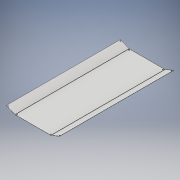
# Autodesk Inventor part: sideplate part 4
Saved by Autodesk Inventor 2018 (Build 220112000, 112)
## iProperties
Created: 2018-06-15
Part Number: sideplate part 4
Material: Generic
Document SubType Name: Sheet Metal
Designer: John Viljoen
Density: 1 g/cm^3
Sheet Metal Rule: Default_mm
Appearance: Default
Flat Pattern Width: 17.41 cm
Flat Pattern Length: 36.287 cm
Flat Pattern Area: 631.755 cm^2
Sheet Metal Width: 174.100 mm
Sheet Metal Length: 362.870 mm
Sheet Metal Area: 63175.525 mm^2
Author: John Viljoen
Autodesk Inventor part; units mm, degrees
ref_plane "YZ Plane" through (0, 0, 0) normal (1, 0, 0) x (0, 1, 0)
ref_plane "XZ Plane" through (0, 0, 0) normal (0, 1, 0) x (-1, 0, 0)
ref_plane "XY Plane" through (0, 0, 0) normal (0, 0, 1) x (1, 0, 0)
sketch "Sketch1" plane through (0, 0, 0) normal (0, 0, 1) x (1, 0, 0)
  line L0 (0, 0) -> (113.5, 0)
  line L1 (113.5, 0) -> (113.5, 338.525)
  line L2 (113.5, 338.525) -> (0, 338.525)
  line L3 (0, 338.525) -> (0, 0)
  dimension "d0" = 113.5
  dimension "d1" = 338.525
  measures "d0" distance of L2.end L1.end
  measures "d1" distance of L1.end L0.end
extrude "Plate1" add sketch "Sketch1" along normal blind 0.5
sketch "Sketch2" plane through (114.0764, 338.525, 0.6152) normal (0.3842953, 0, -0.9232102) x (0, 1, 0)
  line L0 (-338.525, 0) -> (0, 0)
  line L1 (0, 0) -> (0, 29.6214)
  line L2 (0, 29.6214) -> (-338.525, 29.6214)
  line L3 (-338.525, 29.6214) -> (-338.525, 0)
  constraints: 6 end point, 1 horizontal, 1 perpendicular, 1 vertical
edge flange "Flange1" height 30.021 angle 22.6 thickness 0.5 bend radius 1.5 thickness toward (0.3842953, 0, -0.9232102) relief straight relief width 0.5 relief depth 0.25 edges at (113.5, 169.2625, 0.5) wall of the first edge with corners at (114.0764, 0, 0.6152) (114.0764, 338.525, 0.6152) (141.4232, 338.525, 11.9985) (141.4232, 0, 11.9985)
bend "Bend1"
corner "Corner1"
sketch "Sketch3" plane through (-0.5764, 0, 0.6152) normal (-0.3842953, 0, -0.9232102) x (0, -1, 0)
  line L0 (-338.525, 0) -> (0, 0)
  line L1 (0, 0) -> (0, 29.6214)
  line L2 (0, 29.6214) -> (-338.525, 29.6214)
  line L3 (-338.525, 29.6214) -> (-338.525, 0)
  constraints: 6 end point, 1 horizontal, 1 perpendicular, 1 vertical
edge flange "Flange2" height 30.021 angle 22.6 thickness 0.5 bend radius 1.5 thickness toward (-0.3842953, 0, -0.9232102) relief straight relief width 0.5 relief depth 0.25 edges at (0, 169.2625, 0.5) wall of the first edge with corners at (-0.5764, 338.525, 0.6152) (-0.5764, 0, 0.6152) (-27.9232, 0, 11.9985) (-27.9232, 338.525, 11.9985)
bend "Bend2"
corner "Corner2"
sketch "Sketch4" plane through (-27.9232, 0, 11.9985) normal (0.3842953, 0, 0.9232102) x (0.9232102, 0, -0.3842953)
  line L0 (0, 338.525) -> (0, 0) projected
  line L1 (0, 338.525) -> (0, 335.35) construction
  line L2 (0, 335.35) -> (3.175, 335.35) construction
  circle A0 centre (3.175, 335.35) radius 1.25
  line L3 (0, 0) -> (0, 3.175) construction
  line L4 (0, 3.175) -> (3.175, 3.175) construction
  line L5 (3.175, 3.175) -> (3.175, 3.35) construction
  circle A1 centre (3.175, 3.35) radius 1.25
  point P0 (30.39, 0)
  dimension "d23" = 3.175
  dimension "d24" = 3.175
  dimension "d25" = 2.5
  dimension "d26" = 3.175
  dimension "d27" = 3.175
  dimension "d62" = 0.175
  dimension "d63" = 2.5
  constraints: 10 end point, 3 coincident, 2 centre point, 2 perpendicular, 2 point on line, 1 vertical
  measures "d23" distance of L0.start L1.end
  measures "d24" distance of L1.end L2.end
  measures "d25" diameter of A0
  measures "d26" distance of L0.end L3.end
  measures "d27" distance of L3.end L4.end
  measures "d62" distance of L5.start L5.end
  measures "d63" diameter of A1
extrude "Extrusion1" cut sketch "Sketch4" against normal blind 10
sketch "Sketch5" plane through (0, 0, 0.5) normal (0, 0, 1) x (1, 0, 0)
  line L0 (0, 0) -> (0, 338.525) projected
  line L1 (113.5, 0) -> (0, 0) projected
  line L2 (113.5, 338.525) -> (113.5, 0) projected
  line L3 (0, 338.525) -> (0, 335.35) construction
  line L4 (0, 335.35) -> (3.175, 335.35) construction
  line L5 (113.5, 338.525) -> (113.5, 335.35) construction
  line L6 (113.5, 335.35) -> (110.325, 335.35) construction
  line L7 (0, 0) -> (3.175, 0) construction
  line L8 (0, 0) -> (113.5, 0) construction
  line L9 (3.175, 0) -> (3.175, 3.175) construction
  line L10 (113.5, 0) -> (113.5, 3.175) construction
  line L11 (113.5, 3.175) -> (110.325, 3.175) construction
  circle A0 centre (3.175, 335.35) radius 1.25
  circle A1 centre (110.325, 335.35) radius 1.25
  line L12 (3.175, 3.175) -> (3.175, 3.35) construction
  line L13 (110.325, 3.175) -> (110.325, 3.35) construction
  circle A2 centre (110.325, 3.35) radius 1.25
  circle A3 centre (3.175, 3.35) radius 1.25
  dimension "d31" = 3.175
  dimension "d32" = 3.175
  dimension "d33" = 3.175
  dimension "d34" = 3.175
  dimension "d35" = 3.175
  dimension "d36" = 3.175
  dimension "d37" = 3.175
  dimension "d38" = 3.175
  dimension "d41" = 2.5
  dimension "d42" = 2.5
  dimension "d58" = 0.175
  dimension "d59" = 0.175
  dimension "d60" = 2.5
  dimension "d61" = 2.5
  constraints: 20 end point, 6 coincident, 4 centre point, 4 perpendicular, 4 point on line, 2 vertical
  measures "d31" distance of L0.end L3.end
  measures "d32" distance of L3.end L4.end
  measures "d33" distance of L2.start L5.end
  measures "d34" distance of L5.end L6.end
  measures "d35" distance of L0.start L7.end
  measures "d36" distance of L7.end L9.end
  measures "d37" distance of L1.start L10.end
  measures "d38" distance of L10.end L11.end
  measures "d41" diameter of A0
  measures "d42" diameter of A1
  measures "d58" distance of L12.start L12.end
  measures "d59" distance of L13.start L13.end
  measures "d60" diameter of A2
  measures "d61" diameter of A3
extrude "Extrusion2" cut sketch "Sketch5" against normal blind 10
sketch "Sketch6" plane through (141.4232, 0, 11.9985) normal (-0.3842953, 0, 0.9232102) x (0.9232102, 0, 0.3842953)
  line L0 (0, 338.525) -> (0, 335.35) construction
  line L1 (0, 0) -> (0, 338.525) construction
  line L2 (0, 335.35) -> (-3.175, 335.35) construction
  line L3 (0, 0) -> (0, 3.175) construction
  line L4 (0, 3.175) -> (-3.175, 3.175) construction
  circle A0 centre (-3.175, 335.35) radius 1.25
  line L5 (-3.175, 3.175) -> (-3.175, 3.35) construction
  circle A1 centre (-3.175, 3.35) radius 1.25
  point P0 (-135.1743, 0)
  dimension "d45" = 3.175
  dimension "d46" = 3.175
  dimension "d47" = 3.175
  dimension "d48" = 3.175
  dimension "d50" = 2.5
  dimension "d64" = 0.175
  dimension "d65" = 2.5
  constraints: 10 end point, 3 coincident, 2 centre point, 2 perpendicular, 2 point on line, 1 vertical
  measures "d45" distance of L0.start L0.end
  measures "d46" distance of L0.end L2.end
  measures "d47" distance of L1.start L3.end
  measures "d48" distance of L3.end L4.end
  measures "d50" diameter of A0
  measures "d64" distance of L5.start L5.end
  measures "d65" diameter of A1
extrude "Extrusion3" cut sketch "Sketch6" against normal blind 10
sketch "Sketch7" plane through (0, 0, 0.5) normal (0, 0, 1) x (1, 0, 0)
  line L0 (-71.3896, 0) -> (266.456, 0)
  line L1 (266.456, 0) -> (266.456, 0.175)
  line L2 (266.456, 0.175) -> (-71.3896, 0.175)
  line L3 (-71.3896, 0.175) -> (-71.3896, 0)
  dimension "d53" = 0.175
  constraints: 8 end point, 2 parallel, 1 horizontal, 1 perpendicular
  measures "d53" distance of L1.end L0.end
extrude "Extrusion4" cut sketch "Sketch7" against normal blind 100 and the other way blind 100
sketch "Sketch9" plane through (-28.1153, 338.525, 11.5369) normal (0, 1, 0) x (0.9232102, 0, -0.3842953)
  line L0 (29.6214, -0.5) -> (29.6214, 0) projected
  line L1 (29.6214, 0) -> (0, 0) projected
  line L2 (0, -0.5) -> (0, 0) projected
  line L3 (0, -0.5) -> (29.6214, -0.5) projected
  point P0 (30.39, -0.1536)
extrude "Extrusion5" add sketch "Sketch9" along normal blind 30.87
sketch "Sketch10" plane through (0, 338.525, 0.5) normal (0, 1, 0) x (1, 0, 0)
  line L0 (-0.5764, -0.1152) -> (-0.7686, 0.3464) projected
  arc A0 (0, 0) -> (-0.5764, -0.1152) centre (0, -1.5) ccw projected
  line L1 (0, 0.5) -> (0, 0) projected
  arc A1 (0, 0.5) -> (-0.7686, 0.3464) centre (0, -1.5) ccw projected
extrude "Extrusion6" add sketch "Sketch10" along normal blind 30.87
sketch "Sketch11" plane through (0, 338.525, 0) normal (0, 1, 0) x (1, 0, 0)
  line L0 (0, -0.5) -> (113.5, -0.5) projected
  line L1 (113.5, 0) -> (113.5, -0.5) projected
  line L2 (113.5, 0) -> (0, 0) projected
  line L3 (0, 0) -> (0, -0.5) projected
extrude "Extrusion7" add sketch "Sketch11" along normal blind 30.87
sketch "Sketch12" plane through (113.5, 338.525, 0.5) normal (0, 1, 0) x (1, 0, 0)
  line L0 (0.7686, 0.3464) -> (0.5764, -0.1152) projected
  arc A0 (0.7686, 0.3464) -> (0, 0.5) centre (0, -1.5) ccw projected
  line L1 (0, 0.5) -> (0, 0) projected
  arc A1 (0.5764, -0.1152) -> (0, 0) centre (0, -1.5) ccw projected
  point P0 (-113.5, 0.5)
extrude "Extrusion8" add sketch "Sketch12" along normal blind 30.87
sketch "Sketch13" plane through (114.0764, 338.525, 0.6152) normal (0, 1, 0) x (0.9232102, 0, 0.3842953)
  line L0 (0, 0.5) -> (0, 0) projected
  line L1 (29.6214, 0) -> (0, 0) projected
  line L2 (29.6214, 0) -> (29.6214, 0.5) projected
  line L3 (29.6214, 0.5) -> (0, 0.5) projected
  point P0 (-105.553, -43.2711)
extrude "Extrusion9" add sketch "Sketch13" along normal blind 30.87
sketch "Sketch14" plane through (0, 0, 0.5) normal (0, 0, 1) x (1, 0, 0)
  circle A0 centre (3.175, 335.35) radius 1.25 projected
  point P0 (0, 0)
extrude "Extrusion10" add sketch "Sketch14" against normal up to surface (0.5 mm away)
sketch "Sketch15" plane through (0, 0, 0.5) normal (0, 0, 1) x (1, 0, 0)
  circle A0 centre (110.325, 335.35) radius 1.25 projected
  point P0 (0, 0)
extrude "Extrusion11" add sketch "Sketch15" against normal up to surface (0.5 mm away)
sketch "Sketch16" plane through (141.4232, 0.175, 11.9985) normal (-0.3842953, 0, 0.9232102) x (0.9232102, 0, 0.3842953)
  circle A0 centre (-3.175, 335.175) radius 1.25 projected
  point P0 (-135.1743, -0.175)
extrude "Extrusion12" add sketch "Sketch16" against normal up to surface (0.5 mm away)
sketch "Sketch17" plane through (-0.5764, 0.175, 0.6152) normal (0.3842953, 0, 0.9232102) x (0.9232102, 0, -0.3842953)
  circle A0 centre (-26.4464, 335.175) radius 1.25 projected
  point P0 (0.7686, -0.175)
extrude "Extrusion13" add sketch "Sketch17" against normal up to surface (0.5 mm away)
sketch "Sketch18" plane through (0, 0, 0.5) normal (0, 0, 1) x (1, 0, 0)
  line L0 (113.5, 0.175) -> (113.5, 369.395) projected
  line L1 (0, 0.175) -> (0, 369.395) projected
  line L2 (0, 369.395) -> (0, 359.87) construction
  line L3 (0, 359.87) -> (3.175, 359.87) construction
  circle A0 centre (3.175, 359.87) radius 1.5
  line L4 (113.5, 369.395) -> (113.5, 359.87) construction
  line L5 (113.5, 359.87) -> (110.325, 359.87) construction
  circle A1 centre (110.325, 359.87) radius 1.5
  point P0 (0, 0)
  dimension "d84" = 9.525
  dimension "d85" = 3.175
  dimension "d86" = 3
  dimension "d87" = 9.525
  dimension "d88" = 3.175
  dimension "d89" = 3
  constraints: 8 end point, 2 centre point, 2 coincident, 2 perpendicular, 2 point on line
  measures "d84" distance of L1.end L2.end
  measures "d85" distance of L2.end L3.end
  measures "d86" diameter of A0
  measures "d87" distance of L0.end L4.end
  measures "d88" distance of L4.end L5.end
  measures "d89" diameter of A1
extrude "Extrusion14" cut sketch "Sketch18" against normal blind 30.87
sketch "Sketch19" plane through (-0.5764, 0.175, 0.6152) normal (0.3842953, 0, 0.9232102) x (0.9232102, 0, -0.3842953)
  line L0 (-29.6214, 369.22) -> (-29.6214, 0) projected
  line L1 (-29.6214, 369.22) -> (-29.6214, 359.695) construction
  line L2 (-29.6214, 359.695) -> (-26.4464, 359.695) construction
  circle A0 centre (-26.4464, 359.695) radius 1.5
  point P0 (0.7686, -0.175)
  dimension "d92" = 9.525
  dimension "d93" = 3.175
  dimension "d94" = 3
  constraints: 4 end point, 1 centre point, 1 coincident, 1 perpendicular, 1 point on line
  measures "d92" distance of L0.start L1.end
  measures "d93" distance of L1.end L2.end
  measures "d94" diameter of A0
extrude "Extrusion15" cut sketch "Sketch19" against normal blind 30.87
sketch "Sketch20" plane through (141.4232, 0.175, 11.9985) normal (-0.3842953, 0, 0.9232102) x (0.9232102, 0, 0.3842953)
  line L0 (0, 0) -> (0, 369.22) projected
  line L1 (0, 369.22) -> (0, 359.695)
  line L2 (0, 359.695) -> (-3.175, 359.695)
  circle A0 centre (-3.175, 359.695) radius 1.5
  point P0 (-135.1743, -0.175)
  dimension "d97" = 9.525
  dimension "d98" = 3.175
  dimension "d99" = 3
  constraints: 4 end point, 1 centre point, 1 coincident, 1 perpendicular, 1 point on line
  measures "d97" distance of L0.end L1.end
  measures "d98" distance of L1.end L2.end
  measures "d99" diameter of A0
extrude "Extrusion16" cut sketch "Sketch20" against normal blind 30.87
sketch "Sketch21" plane through (0, 0, 0.5) normal (0, 0, 1) x (1, 0, 0)
  line L0 (-35.0424, 369.395) -> (185.2939, 369.395)
  line L1 (185.2939, 369.395) -> (185.2939, 363.045)
  line L2 (185.2939, 363.045) -> (-35.0424, 363.045)
  line L3 (-35.0424, 363.045) -> (-35.0424, 369.395)
  point P0 (0, 0)
  dimension "d102" = 6.35
  constraints: 8 end point, 2 parallel, 1 horizontal, 1 perpendicular
  measures "d102" distance of L0.end L1.end
extrude "Extrusion17" cut sketch "Sketch21" against normal blind 30.87 and the other way blind 15.435
equation "\"d2\" = Thickness"
equation "\"d3\" = BendReliefWidth"
equation "\"d4\" = BendReliefDepth"
equation "\"d5\" = MinimumRemnant"
equation "\"d6\" = TransitionRadius"
equation "\"d10\" = CornerReliefSize"
equation "\"d11\" = GapSize"
equation "\"d12\" = JacobiRadiusSize"
equation "\"d13\" = BendReliefWidth"
equation "\"d14\" = BendReliefDepth"
equation "\"d15\" = MinimumRemnant"
equation "\"d16\" = TransitionRadius"
equation "\"d20\" = CornerReliefSize"
equation "\"d21\" = GapSize"
equation "\"d22\" = JacobiRadiusSize"
equation "\"BendRadius\" = Thickness"
equation "\"BendReliefWidth\" = Thickness"
equation "\"BendReliefDepth\" = 0.5 * Thickness"
equation "\"CornerReliefSize\" = 4 * Thickness"
equation "\"MinimumRemnant\" = 2 * Thickness"
equation "\"TransitionRadius\" = BendRadius"
equation "\"JacobiRadiusSize\" = BendRadius"
equation "\"GapSize\" = Thickness"
equation "\"Thickness\" = 0.5"
body "Solid1"
